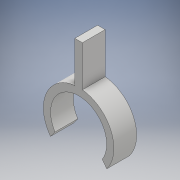
# Autodesk Inventor part: Microphone holder
Saved by Autodesk Inventor 2017 (Build 210142000, 142)
## iProperties
Created: 2018-09-28
Part Number: Microphone holder
Material: Generic
Document SubType Name: Modeling
Designer: Paulius
Density: 1 g/cm^3
Appearance: Default
Author: Paulius
Autodesk Inventor part; units mm, degrees
ref_plane "YZ Plane" through (0, 0, 0) normal (1, 0, 0) x (0, 1, 0)
ref_plane "XZ Plane" through (0, 0, 0) normal (0, 1, 0) x (-1, 0, 0)
ref_plane "XY Plane" through (0, 0, 0) normal (0, 0, 1) x (1, 0, 0)
sketch "Sketch1" plane through (0, 0, 0) normal (0, 1, 0) x (-1, 0, 0)
  arc A0 (3.1129, -2) -> (0, 3.7) centre (0, 0) ccw
  line L0 (3.1129, -2) -> (3.7086, -2.8032)
  arc A1 (3.7086, -2.8032) -> (0.5, 4.6218) centre (0, 0) ccw
  line L1 (0, 10) -> (0.5, 10)
  line L2 (0.5, 10) -> (0.5, 4.6218)
  line L3 (0, 3.7) -> (0, 10)
  arc A2 (0, 3.7) -> (-3.1129, -2) centre (0, 0) ccw
  line L4 (-3.1129, -2) -> (-3.7086, -2.8032)
  arc A3 (-0.5, 4.6218) -> (-3.7086, -2.8032) centre (0, 0) ccw
  line L5 (0, 10) -> (-0.5, 10)
  line L6 (-0.5, 10) -> (-0.5, 4.6218)
  dimension "d0" = 10
  dimension "d1" = 7.4
  dimension "d3" = 1
  dimension "d4" = 0.5
  constraints: 14 end point, 8 point on circle, 4 centre point, 4 symmetric about line, 3 coincident, 2 vertical, 1 horizontal, 2 other
  measures "d0" distance of point (0, 0) L1.start
  measures "d1" diameter of A0
  measures "d3" distance of L0.start L0.end
  measures "d4" distance of L1.start L1.end
extrude "Extrusion1" add sketch "Sketch1" along normal blind 3
body "Solid1"
